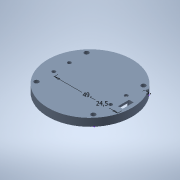
# Autodesk Inventor part: Draaischijf wanden draaischijf
Saved by Autodesk Inventor 2021 (Build 250183000, 183)
## iProperties
Manager: Pierloot J.
Company: Emmaüs Bovenbouw Aalter
Created: 2015-08-18
Part Number: Draaischijf wanden draaischijf
Material: S235
Catalog Web Link: http://emmausbovenbouw.op-weg.be/
Vendor: Emmaüsinstituut Bovenbouw Aalter
Document SubType Name: Modeling
Designer: Pierlootj
Engineer: Pierloot J.
Manufacturer: Standard
Standards Organization: Custom
Density: 7.86 g/cm^3
Appearance: Light Steel Blue
Title: Algemene titel
Subject: Specifieke titel
Author: Pierlootj
Keywords: Ruwe Ø xxxxx
Comments: Opmerking
Autodesk Inventor part; units mm, degrees
ref_plane "YZ Plane" through (0, 0, 0) normal (1, 0, 0) x (0, 1, 0)
ref_plane "XZ Plane" through (0, 0, 0) normal (0, 1, 0) x (-1, 0, 0)
ref_plane "XY Plane" through (0, 0, 0) normal (0, 0, 1) x (1, 0, 0)
sketch "Sketch14" plane through (0, 0, 0) normal (0, 0, 1) x (1, 0, 0)
  line L0 (0, 0) -> (-24.5, 0)
  line L1 (-24.5, 0) -> (24.5, 0)
  circle A0 centre (0, 0) radius 32.5
  line L2 (-24.5, 0) -> (-24.5, -21.354157)
  line L3 (-24.5, 21.354157) -> (-19.5, 21.354157)
  line L4 (-19.5, 21.354157) -> (-19.5, -21.354157)
  line L5 (-19.5, -21.354157) -> (-24.5, -21.354157)
  line L6 (-24.5, -21.354157) -> (-24.5, 21.354157)
  line L7 (0, 27.066827) -> (0, -27.008994)
  line L8 (24.5, 21.354157) -> (19.5, 21.354157)
  line L9 (19.5, 21.354157) -> (19.5, -21.354157)
  line L10 (19.5, -21.354157) -> (24.5, -21.354157)
  line L11 (24.5, -21.354157) -> (24.5, 21.354157)
  dimension "d105" = 24.5
  dimension "d106" = 49
  dimension "d107" = 65
  dimension "d108" = 5
  constraints: 24 end point, 4 symmetric about line, 2 horizontal, 2 parallel, 2 point on circle, 2 vertical, 1 centre point, 1 coincident, 1 perpendicular, 1 point on line
  measures "d105" distance of L0.start L0.end
  measures "d106" distance of L0.end L1.end
  measures "d107" diameter of A0
  measures "d108" distance of L4.end L5.end
extrude "Extrusion12" add sketch "Sketch14" along normal blind 6
sketch "Sketch15" plane through (0, 0, 6) normal (0, 0, 1) x (1, 0, 0)
  line L0 (0, 0) -> (-24.5, 0)
  line L1 (-24.5, 0) -> (24.5, 0)
  line L2 (-24.5, -21.354157) -> (-24.5, 21.354157)
  line L3 (0, 27.066827) -> (0, -27.008994)
  line L4 (19.5, -21.354157) -> (24.5, -21.354157)
  line L5 (19.5, 21.354157) -> (19.5, -21.354157)
  line L6 (24.5, -21.354157) -> (24.5, 21.354157)
  line L7 (24.5, 21.354157) -> (19.5, 21.354157)
  line L8 (-24.5, -21.354157) -> (-19.5, -21.354157)
  line L9 (-19.5, -21.354157) -> (-19.5, 21.354157)
  line L10 (-19.5, 21.354157) -> (-24.5, 21.354157)
  line L11 (-24.5, 21.354157) -> (-24.5, -21.354157)
  dimension "d111" = 24.5
  dimension "d112" = 49
  dimension "d131" = 5
  constraints: 24 end point, 2 horizontal, 2 parallel, 2 symmetric about line, 1 perpendicular, 1 point on line, 1 vertical
  measures "d111" distance of L0.start L0.end
  measures "d112" distance of L0.end L1.end
  measures "d131" distance of L10.end L9.end
extrude "Extrusion13" add sketch "Sketch15" along normal blind 50
fillet "Fillet5" radius 21.3 2 edges at (22, -21.3542, 56) (22, 21.3542, 56)
sketch "Sketch17" plane through (24.5, -21.354157, 6) normal (1, 0, 0) x (0, 0, -1)
  line L0 (0, 42.708313) -> (0, 0)
  line L1 (0, 21.354157) -> (-30, 21.354157)
  line L2 (-30, 21.354157) -> (-13.35, 21.354157)
  line L3 (-13.35, 21.354157) -> (-13.35, 27.509236)
  line L4 (-13.35, 27.509236) -> (-36.15, 27.509236)
  line L5 (-36.15, 27.509236) -> (-36.15, 15.209236)
  line L6 (-36.15, 15.209236) -> (-13.35, 15.209236)
  line L7 (-13.35, 15.209236) -> (-13.35, 27.509236)
  point P0 (6, 21.354157)
  dimension "d122" = 30
  dimension "d190" = 16.65
  dimension "d191" = 22.8
  dimension "d192" = 12.3
  constraints: 14 end point, 2 horizontal, 2 parallel, 2 perpendicular, 1 midpoint, 1 point on line
  measures "d122" distance of L1.start L1.end
  measures "d190" distance of L1.end L2.end
  measures "d191" distance of L6.end L5.end
  measures "d192" distance of L5.end L4.end
sketch "Sketch19" plane through (-24.5, -21.354157, 6) normal (-1, 0, 0) x (0, 0, 1)
  line L0 (0, 0) -> (0, 42.708313)
  line L1 (0, 21.354157) -> (30, 21.354157)
  circle A0 centre (30, 21.354157) radius 7.65
  point P0 (-6, 21.354157)
  dimension "d132" = 30
  dimension "d184" = 15.3
  constraints: 2 end point, 1 centre point, 1 coincident, 1 horizontal, 1 midpoint
  measures "d132" distance of L1.start L1.end
  measures "d184" diameter of A0
fillet "Fillet6" radius 21.3 2 edges at (-22, 21.3542, 56) (-22, -21.3542, 56)
sketch "Sketch20" plane through (-24.5, -21.354157, 6) normal (-1, 0, 0) x (0, 0, 1)
  circle A0 centre (30, 21.354157) radius 13
  circle A1 centre (30, 21.354157) radius 6.5
  circle A2 centre (30, 21.354157) radius 7.75
  point P0 (-6, 21.354157)
  dimension "d137" = 13
  dimension "d138" = 15.5
  constraints: 2 centre point, 2 coincident
  measures "d137" diameter of A1
  measures "d138" diameter of A2
extrude "Extrusion18" add sketch "Sketch20" along normal blind 1 contours A2
sketch "Sketch21" plane through (0, 0, 0) normal (0, 0, -1) x (-1, 0, 0)
  circle A0 centre (0, 0) radius 2.5 projected
  circle A1 centre (0, 0) radius 26.15
  circle A2 centre (0, 0) radius 17.35
  dimension "d144" = 52.3
  dimension "d145" = 34.7
  constraints: 2 centre point, 2 coincident
  measures "d144" diameter of A1
  measures "d145" diameter of A2
extrude "Extrusion19" cut sketch "Sketch21" against normal blind 4.3 contours A1
sketch "Sketch22" plane through (24.5, -21.354157, 6) normal (1, 0, 0) x (0, 0, -1)
  point P0 (6, 21.354157)
sketch "Sketch23" plane through (24.5, -21.354157, 6) normal (1, 0, 0) x (0, 0, -1)
  line L0 (-35.75, 27.504157) -> (-35.75, 15.204157)
  line L1 (-35.75, 21.354157) -> (-38.25, 21.354157)
  circle A0 centre (-38.25, 21.354157) radius 0.5
  line L2 (-13.25, 27.504157) -> (-13.25, 15.204157)
  line L3 (-13.25, 21.354157) -> (-11.25, 21.354157)
  circle A1 centre (-11.25, 21.354157) radius 0.5
  point P0 (6, 21.354157)
  dimension "d150" = 2.5
  dimension "d151" = 1
  dimension "d152" = 2
  dimension "d153" = 1
  constraints: 4 end point, 2 centre point, 2 coincident, 2 horizontal, 2 midpoint
  measures "d150" distance of L1.start L1.end
  measures "d151" diameter of A0
  measures "d152" distance of L3.start L3.end
  measures "d153" diameter of A1
extrude "Extrusion21" cut sketch "Sketch23" against normal up to surface (5 mm away)
extrude "Extrusion23" cut sketch "Sketch19" against normal up to surface (5 mm away)
chamfer "Chamfer2" distance 1 angle 45 1 edges at (-24.5, 0, 28.25)
extrude "Extrusion24" cut sketch "Sketch17" against normal up to surface (5 mm away)
sketch "Sketch25" plane through (0, 0, 0) normal (0, 0, -1) x (-1, 0, 0)
  arc A0 (2.196942, 15.215949) -> (-2.196942, 15.215949) centre (0, 15.1) ccw
  line L0 (2.196942, 15.215949) -> (2.899204, 1.909835)
  line L1 (-2.196942, 15.215949) -> (-2.89394, 2.009577)
  line L2 (2.899204, 1.909835) -> (3, 0) construction
  line L3 (-2.89394, 2.009577) -> (-3, 0) construction
  line L4 (-13.697938, 0) -> (13.243784, 0) construction
  line L5 (2.196942, -15.215949) -> (2.899204, -1.909835)
  line L6 (-2.196942, -15.215949) -> (-2.89394, -2.009577)
  arc A1 (-2.196942, -15.215949) -> (2.196942, -15.215949) centre (0, -15.1) ccw
  line L7 (-2.89394, -2.009577) -> (-3, 0) construction
  line L8 (2.899204, -1.909835) -> (3, 0) construction
  arc A2 (7.35, -1.1) -> (7.35, 1.1) centre (7.35, 0) ccw
  arc A3 (-7.35, 1.1) -> (-7.387068, -1.099375) centre (-7.35, 0) ccw
  arc A4 (2.899204, -1.909835) -> (3.206651, -1.1) centre (-0.228741, -0.25906) ccw
  arc A5 (3.326692, 1.1) -> (2.899204, 1.909835) centre (-0.228741, -0.25906) ccw
  arc A6 (-2.89394, 2.009577) -> (-3.454102, 1.1) centre (-0.228741, -0.25906) ccw
  arc A7 (-3.263283, -1.23842) -> (-2.89394, -2.009577) centre (-0.228741, -0.25906) ccw
  line L9 (7.35, 1.1) -> (3.326692, 1.1)
  line L10 (-3.454102, 1.1) -> (-7.35, 1.1)
  line L11 (7.35, -1.1) -> (3.206651, -1.1)
  line L12 (-3.263283, -1.23842) -> (-7.387068, -1.099375)
  line L13 (-3.875949, 2.376821) -> (-3.195553, 15.268653)
  line L14 (3.195553, 15.268653) -> (3.883777, 2.228509)
  arc A8 (3.958817, 2.1) -> (3.883777, 2.228509) centre (-0.228741, -0.25906) ccw
  line L15 (3.958817, 2.1) -> (7.35, 2.1)
  arc A9 (7.35, -2.1) -> (7.35, 2.1) centre (7.35, 0) ccw
  line L16 (7.35, -2.1) -> (3.917785, -2.1)
  arc A10 (3.886977, -2.167883) -> (3.917785, -2.1) centre (-0.228741, -0.25906) ccw
  line L17 (3.886977, -2.167883) -> (3.195553, -15.268653)
  line L18 (-3.195553, -15.268653) -> (-3.879324, -2.312878)
  arc A11 (-3.931926, -2.216443) -> (-3.879324, -2.312878) centre (-0.228741, -0.25906) ccw
  line L19 (-3.931926, -2.216443) -> (-7.420767, -2.098807)
  arc A12 (-7.35, 2.1) -> (-7.420767, -2.098807) centre (-7.35, 0) ccw
  line L20 (-7.35, 2.1) -> (-4.06082, 2.1)
  arc A13 (-3.875949, 2.376821) -> (-4.06082, 2.1) centre (-0.228741, -0.25906) ccw
  circle A14 centre (0, 0) radius 17.35
  arc A15 (2.433021, 17.17856) -> (-2.433021, 17.17856) centre (0, 0) ccw
  arc A16 (-2.433021, -17.17856) -> (2.433021, -17.17856) centre (0, 0) ccw
  arc A17 (3.195553, 15.268653) -> (2.433021, 17.17856) centre (0, 15.1) ccw
  arc A18 (-2.433021, 17.17856) -> (-3.195553, 15.268653) centre (0, 15.1) ccw
  arc A19 (-3.195553, -15.268653) -> (-2.433021, -17.17856) centre (0, -15.1) ccw
  arc A20 (2.433021, -17.17856) -> (3.195553, -15.268653) centre (0, -15.1) ccw
  dimension "d197" = 3
  dimension "d198" = 3
  dimension "d199" = 15.1
  dimension "d200" = 2.2
  dimension "d201" = 2.2
  dimension "d202" = 2.2
  dimension "d203" = 14.7
  dimension "d204" = 7.35
  dimension "d205" = 1
  constraints: 44 point on circle, 42 end point, 20 centre point, 6 tangent, 5 symmetric about line, 3 point on line, 2 coincident, 2 horizontal alignment, 2 parallel, 1 horizontal, 1 vertical alignment, 12 other
  measures "d197" distance of L2.end point (0, 0)
  measures "d198" distance of L3.end point (0, 0)
  measures "d199" distance of A0.centre point (0, 0)
  measures "d200" radius of A0
  measures "d201" diameter of A2
  measures "d202" diameter of A3
  measures "d203" distance of A3.centre A2.centre
  measures "d204" distance of point (0, 0) A2.centre
  measures "d205" distance between parallel lines of L1 L13
extrude "Extrusion26" add sketch "Sketch25" along normal blind 2.6 contours L13 A18 A14 A17 L14 A8 L15 A9 L16 A10 L17 A20 A19 L18 A11 L19 A12 L20 A13
chamfer "Chamfer3" distance 1 angle 45 11 edges at (3.5374, -8.7908, 0) (2.9719, -16.2865, 0) (5.6763, -2.1576, 0) (9.4497, 0.0354, 0) (5.7054, 2.1, 0) (3.5358, 8.8227, 0) (2.9719, 16.2865, 0) (-3.5413, -8.7183, 0) (-2.9719, -16.2865, 0) (-3.5397, 8.7486, 0) (-2.9719, 16.2865, 0)
sketch "Sketch26" plane through (0, 0, -2.6) normal (0, 0, -1) x (-1, 0, 0)
  arc A0 (3.778648, -16.933526) -> (3.778648, 16.933526) centre (0, 0) ccw
  arc A1 (-3.778648, 16.933526) -> (-3.778648, -16.933526) centre (0, 0) ccw
  arc A2 (5.256809, 16.534463) -> (-4.669618, 16.709793) centre (0, 0) ccw
  arc A3 (4.60866, 15.687025) -> (-4.498174, 15.719063) centre (0, 0) ccw
  line L0 (-4.669618, 16.709793) -> (-4.498174, 15.719063)
  line L1 (4.60866, 15.687025) -> (5.256809, 16.534463)
  line L2 (-13.837791, 0) -> (14.489544, 0)
  arc A4 (-4.669618, -16.709793) -> (5.256809, -16.534463) centre (0, 0) ccw
  arc A5 (-4.498174, -15.719063) -> (4.60866, -15.687025) centre (0, 0) ccw
  line L3 (-4.669618, -16.709793) -> (-4.498174, -15.719063)
  line L4 (4.60866, -15.687025) -> (5.256809, -16.534463)
  point P0 (-3.778648, -16.933526)
  point P1 (3.778648, 16.933526)
  dimension "d211" = 16.35
  constraints: 10 end point, 10 point on circle, 4 centre point, 4 symmetric about line, 2 coincident, 1 horizontal, 2 other
  measures "d211" radius of A3
extrude "Extrusion27" cut sketch "Sketch26" against normal blind 2.6 contours A4 A1 L3 A5 L4 A0 | L1 A3 L0 A1 A2 A0
sketch "Sketch29" plane through (0, 0, 6) normal (0, 0, 1) x (1, 0, 0)
  line L0 (24.5, 21.354157) -> (24.5, -21.354157)
  line L1 (24.5, 0) -> (26, 0)
  line L2 (26, 0) -> (26, 4.25)
  line L3 (26, 4.25) -> (29.5, 4.25)
  line L4 (29.5, 4.25) -> (29.5, -4.25)
  line L5 (29.5, -4.25) -> (26, -4.25)
  line L6 (26, -4.25) -> (26, 4.25)
  point P0 (0, 0)
  dimension "d226" = 1.5
  dimension "d227" = 4.25
  dimension "d228" = 3.5
  dimension "d229" = 8.5
  constraints: 12 end point, 2 horizontal, 2 parallel, 2 perpendicular, 1 midpoint
  measures "d226" distance of L1.start L1.end
  measures "d227" distance of L1.end L2.end
  measures "d228" distance of L4.end L5.end
  measures "d229" distance of L3.end L4.end
extrude "Extrusion30" cut sketch "Sketch29" against normal through all
sketch "Sketch30" plane through (0, 0, 6) normal (0, 0, 1) x (1, 0, 0)
  circle A0 centre (0, 0) radius 52.166379
  constraints: 1 centre point, 1 coincident
extrude "Extrusion31" cut sketch "Sketch30" along normal blind 56.75
sketch "Sketch31" plane through (0, 0, 6) normal (0, 0, 1) x (1, 0, 0)
  line L0 (0, 0) -> (-24.5, 0)
  line L1 (-24.5, 0) -> (24.5, 0)
  line L2 (-24.5, -21.354157) -> (-24.5, 21.354157)
  line L3 (0, 27.066827) -> (0, -27.008994)
  line L4 (19.5, -21.354157) -> (24.5, -21.354157)
  line L5 (19.5, 21.354157) -> (19.5, -21.354157)
  line L6 (24.5, -21.354157) -> (24.5, 21.354157)
  line L7 (24.5, 21.354157) -> (19.5, 21.354157)
  line L8 (-24.5, -21.354157) -> (-19.5, -21.354157)
  line L9 (-19.5, -21.354157) -> (-19.5, 21.354157)
  line L10 (-19.5, 21.354157) -> (-24.5, 21.354157)
  line L11 (-24.5, 21.354157) -> (-24.5, -21.354157)
  line L12 (19.5, 0) -> (22, 0)
  line L13 (22, 0) -> (22, 6)
  line L14 (22, 6) -> (22, -6)
  circle A0 centre (22, 6) radius 1.35
  circle A1 centre (22, -6) radius 1.35
  line L15 (0, 0) -> (0, 8.717276)
  circle A2 centre (-22, 6) radius 1.35
  circle A3 centre (-22, -6) radius 1.35
  dimension "d234" = 24.5
  dimension "d235" = 49
  dimension "d236" = 5
  dimension "d243" = 2.5
  dimension "d244" = 6
  dimension "d245" = 12
  dimension "d246" = 2.7
  dimension "d247" = 2.7
  constraints: 32 end point, 4 centre point, 4 point on line, 4 symmetric about line, 2 coincident, 2 horizontal, 2 parallel, 2 perpendicular, 1 midpoint, 1 vertical, 2 other
  measures "d234" distance of L0.start L0.end
  measures "d235" distance of L0.end L1.end
  measures "d236" distance of L10.end L9.end
  measures "d243" distance of L12.start L12.end
  measures "d244" distance of L12.end L13.end
  measures "d245" distance of L13.end L14.end
  measures "d246" diameter of A0
  measures "d247" diameter of A1
sketch "Sketch32" plane through (0, 0, 0) normal (0, 0, -1) x (-1, 0, 0)
  line L0 (0, 0) -> (-24.5, 0)
  line L1 (-24.5, 0) -> (24.5, 0)
  line L2 (-24.5, -21.354157) -> (-24.5, 21.354157)
  line L3 (0, 27.066827) -> (0, -27.008994)
  line L4 (19.5, -21.354157) -> (24.5, -21.354157)
  line L5 (19.5, 21.354157) -> (19.5, -21.354157)
  line L6 (24.5, -21.354157) -> (24.5, 21.354157)
  line L7 (24.5, 21.354157) -> (19.5, 21.354157)
  line L8 (-24.5, -21.354157) -> (-19.5, -21.354157)
  line L9 (-19.5, -21.354157) -> (-19.5, 21.354157)
  line L10 (-19.5, 21.354157) -> (-24.5, 21.354157)
  line L11 (-24.5, 21.354157) -> (-24.5, -21.354157)
  dimension "d237" = 24.5
  dimension "d238" = 49
  dimension "d239" = 5
  constraints: 24 end point, 2 horizontal, 2 parallel, 2 symmetric about line, 1 perpendicular, 1 point on line, 1 vertical
  measures "d237" distance of L0.start L0.end
  measures "d238" distance of L0.end L1.end
  measures "d239" distance of L10.end L9.end
sketch "Sketch33" plane through (0, 0, 0) normal (0, 0, -1) x (-1, 0, 0)
  circle A0 centre (0, 0) radius 32.5
  line L0 (-24.500005, -21.354151) -> (-19.500077, -17.423245)
  arc A1 (-26, -2.796873) -> (-26, 2.796873) centre (0, 0) ccw
  line L1 (-19.500077, -17.423245) -> (-22.000041, -19.388698)
  circle A2 centre (-22.000041, -19.388698) radius 1.75
  line L2 (0, 0) -> (-22.866569, 0)
  circle A3 centre (-22.000041, 19.388698) radius 1.75
  line L3 (0, -23.308415) -> (0, 14.949616)
  circle A4 centre (22.000041, -19.388698) radius 1.75
  circle A5 centre (22.000041, 19.388698) radius 1.75
  dimension "d240" = 3.5
  constraints: 8 end point, 4 centre point, 3 symmetric about line, 1 coincident, 1 horizontal, 1 midpoint, 1 point on circle, 1 vertical, 5 other
  measures "d240" diameter of A2
extrude "Extrusion32" cut sketch "Sketch33" against normal through all contours A2 L0 | L0 A2 | A3 | A4 | A5
extrude "Extrusion33" cut sketch "Sketch31" against normal through all contours A0 | A1 | A2 | A3
body "Solid6"
